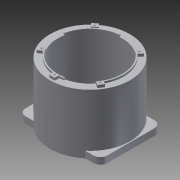
# Autodesk Inventor part: F-mount to CMV12k-V04
Saved by Autodesk Inventor 2015 (Build 190159000, 159)
## iProperties
Created: 2012-09-30
Part Number: F-mount to CMV12k-V04
Document SubType Name: Modeling
Designer: ko
Density: 2.71 g/cm^3
Material: Aluminum-6061
Mass: 114.122 g
Surface Area: 182.607 cm^2
Volume: 42.1113 cm^3
Appearance: Aluminum - Flat
Author: ko
Autodesk Inventor part; units mm, degrees
ref_plane "YZ Plane" through (0, 0, 0) normal (1, 0, 0) x (0, 1, 0)
ref_plane "XZ Plane" through (0, 0, 0) normal (0, 1, 0) x (-1, 0, 0)
ref_plane "Work Plane2" through (0, 0, -4.13) normal (0, 0, 1) x (1, 0, 0)
ref_plane "F-mount flange back plane" through (0, 0, -2.23) normal (0, 0, 1) x (1, 0, 0)
sketch "Sketch2" plane through (0, 0, -4.13) normal (0, 0, 1) x (1, 0, 0)
  circle A0 centre (0, 0) radius 29
  dimension "d2" = 58
  constraints: 1 centre point, 1 coincident
  measures "d2" diameter of A0
sketch "Sketch4" plane through (0, 0, 0) normal (0, 1, 0) x (-1, 0, 0)
  line L0 (0, 0) -> (0, -97.328378) construction
  arc A0 (92.740295, -62.593615) -> (0, 0) centre (0, -100) ccw
  line L1 (29, -4.13) -> (-29, -4.13)
  dimension "d19" = 100
  constraints: 2 end point, 2 point on circle, 1 centre point, 1 point on line, 1 vertical, 2 other
  measures "d19" distance of L0.start A0.centre
ref_plane "Focal plane" through (0, 0, -46.5) normal (0, 0, 1) x (1, 0, 0)
ref_plane "Back origin" through (0, 0, -47.25) normal (0, 0, 1) x (1, 0, 0)
sketch "Sketch3" plane through (0, 0, -46.5) normal (0, 0, 1) x (1, 0, 0)
  line L0 (-24.3, -16.9) -> (22.7, -16.9) construction
  line L1 (22.7, 16.9) -> (-24.3, 16.9) construction
  line L2 (-12.6, 11.4) -> (12.6, 11.4) construction
  line L3 (12.6, 11.4) -> (12.6, -11.4) construction
  line L4 (12.6, -11.4) -> (-12.6, -11.4) construction
  line L5 (-12.6, -11.4) -> (-12.6, 11.4) construction
  line L6 (47.757602, 0) -> (-47.757602, 0) construction
  line L7 (0, 37.75526) -> (0, -37.75526) construction
  line L8 (-0.8, 20.026863) -> (-0.8, -19.024317) construction
  line L9 (22.7, 1.75) -> (20.7, 1.75) construction
  line L10 (20.7, -1.75) -> (22.7, -1.75) construction
  arc A0 (20.7, 1.75) -> (20.7, -1.75) centre (20.7, 0) ccw construction
  line L11 (22.7, 8.9) -> (18.7, 8.9) construction
  line L12 (18.7, 8.9) -> (18.7, 12.9) construction
  line L13 (18.7, 12.9) -> (22.7, 12.9) construction
  line L14 (22.7, 1.75) -> (22.7, 8.9) construction
  line L15 (22.7, 12.9) -> (22.7, 16.9) construction
  line L16 (22.7, -8.9) -> (18.7, -8.9) construction
  line L17 (18.7, -8.9) -> (18.7, -12.9) construction
  line L18 (18.7, -12.9) -> (22.7, -12.9) construction
  line L19 (22.7, -1.75) -> (22.7, -8.9) construction
  line L20 (22.7, -12.9) -> (22.7, -16.9) construction
  line L21 (-24.3, 1.75) -> (-22.3, 1.75) construction
  line L22 (-22.3, -1.75) -> (-24.3, -1.75) construction
  arc A1 (-22.3, -1.75) -> (-22.3, 1.75) centre (-22.3, 0) ccw construction
  line L23 (-24.3, 8.9) -> (-20.3, 8.9) construction
  line L24 (-20.3, 8.9) -> (-20.3, 12.9) construction
  line L25 (-20.3, 12.9) -> (-24.3, 12.9) construction
  line L26 (-24.3, 1.75) -> (-24.3, 8.9) construction
  line L27 (-24.3, 12.9) -> (-24.3, 16.9) construction
  line L28 (-20.3, -8.9) -> (-20.3, -12.9) construction
  line L29 (-24.3, -12.9) -> (-24.3, -16.9) construction
  line L30 (-20.3, -12.9) -> (-24.3, -12.9) construction
  line L31 (-24.3, -8.9) -> (-20.3, -8.9) construction
  line L32 (-24.3, -1.75) -> (-24.3, -8.9) construction
  line L33 (-20.198295, -17.2) -> (-20.43657, -17.382277)
  line L34 (-24.65, -22.15) -> (24.65, -22.15)
  line L35 (29.65, -17.15) -> (29.65, 17.15)
  line L36 (24.65, 22.15) -> (-24.65, 22.15)
  line L37 (-29.65, 17.15) -> (-29.65, -17.15)
  arc A2 (29.65, 17.15) -> (24.65, 22.15) centre (24.65, 17.15) ccw
  arc A3 (24.65, -22.15) -> (29.65, -17.15) centre (24.65, -17.15) ccw
  arc A4 (-29.65, -17.15) -> (-24.65, -22.15) centre (-24.65, -17.15) ccw
  arc A5 (-24.65, 22.15) -> (-29.65, 17.15) centre (-24.65, 17.15) ccw
  line L38 (-24.238989, 12.5) -> (-28.238989, 12.5) construction
  line L39 (-24.3, 12.9) -> (-29.65, 12.9) construction
  line L40 (-27.5, 13.045808) -> (-27.5, 9.045808) construction
  line L41 (28.625588, -12.5) -> (20.569896, -12.5) construction
  line L42 (27.5, -9.401134) -> (27.5, -14.475126) construction
  line L43 (-18.15, 16.9) -> (16.55, 16.9) construction
  line L44 (16.55, 16.9) -> (16.55, -16.9) construction
  line L45 (16.55, -16.9) -> (-18.15, -16.9) construction
  line L46 (-18.15, -16.9) -> (-18.15, 16.9) construction
  point P0 (0, 0)
  point P1 (0, 0)
  point P2 (0, 0)
  point P3 (-20.3, 10.9)
  point P4 (-27.5, 12.5)
  point P5 (27.5, -12.5)
  dimension "d5" = 16.9
  dimension "d6" = 47
  dimension "d7" = 33.8
  dimension "d8" = 25.2
  dimension "d9" = 22.8
  dimension "d10" = 3.5
  dimension "d11" = 2
  dimension "d12" = 4
  dimension "d13" = 4
  dimension "d14" = 4
  dimension "d15" = 24.3
  dimension "d135" = 59.3
  dimension "d136" = 44.3
  dimension "d137" = 5
  dimension "d164" = 55
  dimension "d165" = 25
  dimension "d169" = 34.7
  dimension "d170" = 0
  dimension "d171" = 0
  dimension "d172" = 6.15
  dimension "d173" = 6.2
  constraints: 94 end point, 17 symmetric about line, 12 point on circle, 10 tangent, 9 parallel, 6 centre point, 5 perpendicular, 5 vertical, 4 collinear, 4 horizontal, 4 point on line, 3 equal radius, 3 midpoint, 2 coincident, 8 other
  measures "d5" distance from line of point (0, 0) L0
  measures "d6" distance of L1.start L1.end
  measures "d7" distance of L0.end L1.start
  measures "d8" distance of L2.start L2.end
  measures "d9" distance of L2.end L3.end
  measures "d10" distance between parallel lines of L10 L9
  measures "d11" distance of L9.start L9.end
  measures "d12" distance of L11.end L12.end
  measures "d13" distance of L12.end L13.end
  measures "d14" distance between parallel lines of L1 L13
  measures "d15" distance from line of L7 L0.start
  measures "d135" distance between parallel lines of L37 L35
  measures "d136" distance between parallel lines of L34 L36
  measures "d137" radius of A2
  measures "d164" distance between parallel lines of L42 L40
  measures "d165" distance between parallel lines of L38 L41
  measures "d169" distance of L43.start L43.end
  measures "d170" distance between parallel lines of L0 L45
  measures "d171" distance between parallel lines of L1 L43
  measures "d172" distance between parallel lines of L27 L46
sketch "Sketch6" plane through (0, 0, -46.5) normal (0, 0, 1) x (1, 0, 0)
  line L0 (-0.8, 17.2) -> (-24.3, 17.2)
  line L1 (22.7, 16.9) -> (-24.3, 16.9) construction
  line L2 (-24.3, 12.9) -> (-24.3, 16.9) construction
  arc A0 (-24.3, 17.2) -> (-24.3, 12.775) centre (-24.3, 14.9875) ccw
  line L3 (47.757602, 0) -> (-47.757602, 0) construction
  line L4 (-0.8, 20.026863) -> (-0.8, -19.024317) construction
  line L5 (22.7, 16.9) -> (22.912132, 17.112132) construction
  line L6 (-24.3, 12.775) -> (-20.925, 12.775)
  line L7 (-20.425, 12.275) -> (-20.425, 9.525)
  line L8 (-20.925, 9.025) -> (-24.3, 9.025)
  line L9 (-20.3, 12.9) -> (-24.3, 12.9) construction
  line L10 (-20.3, 8.9) -> (-20.3, 12.9) construction
  line L11 (-24.3, 8.9) -> (-20.3, 8.9) construction
  line L12 (-26.5125, 0) -> (-26.5125, 6.8125)
  arc A1 (-24.3, 9.025) -> (-26.5125, 6.8125) centre (-24.3, 6.8125) ccw
  arc A2 (-20.425, 12.275) -> (-20.925, 12.775) centre (-20.925, 12.275) ccw
  arc A3 (-20.925, 9.025) -> (-20.425, 9.525) centre (-20.925, 9.525) ccw
  line L13 (-0.8, -17.2) -> (-24.3, -17.2)
  line L14 (22.7, -16.9) -> (-24.3, -16.9) construction
  line L15 (-24.3, -12.9) -> (-24.3, -16.9) construction
  arc A4 (-24.3, -12.775) -> (-24.3, -17.2) centre (-24.3, -14.9875) ccw
  line L16 (-24.3, -12.775) -> (-20.925, -12.775)
  line L17 (-20.425, -12.275) -> (-20.425, -9.525)
  line L18 (-20.925, -9.025) -> (-24.3, -9.025)
  line L19 (-20.3, -12.9) -> (-24.3, -12.9) construction
  line L20 (-20.3, -8.9) -> (-20.3, -12.9) construction
  line L21 (-24.3, -8.9) -> (-20.3, -8.9) construction
  line L22 (-26.5125, 0) -> (-26.5125, -6.8125)
  arc A5 (-26.5125, -6.8125) -> (-24.3, -9.025) centre (-24.3, -6.8125) ccw
  arc A6 (-20.925, -12.775) -> (-20.425, -12.275) centre (-20.925, -12.275) ccw
  arc A7 (-20.425, -9.525) -> (-20.925, -9.025) centre (-20.925, -9.525) ccw
  line L23 (-0.8, 17.2) -> (22.7, 17.2)
  line L24 (-24.3, 16.9) -> (22.7, 16.9) construction
  line L25 (22.7, 12.9) -> (22.7, 16.9) construction
  arc A8 (22.7, 12.775) -> (22.7, 17.2) centre (22.7, 14.9875) ccw
  line L26 (-49.357602, 0) -> (46.157602, 0) construction
  line L27 (22.7, 12.775) -> (19.325, 12.775)
  line L28 (18.825, 12.275) -> (18.825, 9.525)
  line L29 (19.325, 9.025) -> (22.7, 9.025)
  line L30 (18.7, 12.9) -> (22.7, 12.9) construction
  line L31 (18.7, 8.9) -> (18.7, 12.9) construction
  line L32 (22.7, 8.9) -> (18.7, 8.9) construction
  line L33 (24.9125, 0) -> (24.9125, 6.8125)
  arc A9 (24.9125, 6.8125) -> (22.7, 9.025) centre (22.7, 6.8125) ccw
  arc A10 (19.325, 12.775) -> (18.825, 12.275) centre (19.325, 12.275) ccw
  arc A11 (18.825, 9.525) -> (19.325, 9.025) centre (19.325, 9.525) ccw
  line L34 (22.7, -12.9) -> (22.7, -16.9) construction
  line L35 (18.7, -8.9) -> (18.7, -12.9) construction
  line L36 (18.825, -12.275) -> (18.825, -9.525)
  arc A12 (18.825, -12.275) -> (19.325, -12.775) centre (19.325, -12.275) ccw
  arc A13 (19.325, -9.025) -> (18.825, -9.525) centre (19.325, -9.525) ccw
  line L37 (18.7, -12.9) -> (22.7, -12.9) construction
  line L38 (22.7, -8.9) -> (18.7, -8.9) construction
  line L39 (19.325, -9.025) -> (22.7, -9.025)
  line L40 (22.7, -12.775) -> (19.325, -12.775)
  arc A14 (22.7, -17.2) -> (22.7, -12.775) centre (22.7, -14.9875) ccw
  line L41 (24.9125, 0) -> (24.9125, -6.8125)
  arc A15 (22.7, -9.025) -> (24.9125, -6.8125) centre (22.7, -6.8125) ccw
  line L42 (-0.8, -17.2) -> (22.7, -17.2)
  line L43 (-24.3, -16.9) -> (22.7, -16.9) construction
  point P0 (0, 0)
  point P1 (-0.8, -20.026863)
  dimension "d37" = 0.3
  dimension "d41" = 0.125
  dimension "d42" = 0.125
  dimension "d43" = 0.125
  dimension "d45" = 2.2125
  dimension "d47" = 0.5
  constraints: 74 end point, 59 symmetric about line, 32 point on circle, 16 centre point, 11 point on line, 8 tangent, 2 equal radius, 1 parallel, 12 other
  measures "d37" distance between parallel lines of L1 L0
  measures "d41" distance between parallel lines of L6 L9
  measures "d42" distance between parallel lines of L10 L7
  measures "d43" distance between parallel lines of L11 L8
  measures "d45" radius of A0
  measures "d47" radius of A2
sketch "Sketch5" plane through (0, 0, -4.13) normal (0, 0, 1) x (1, 0, 0)
  line L0 (29.3063, -36.610535) -> (-29.3063, -36.610535)
  line L1 (-39.3063, -26.610535) -> (-39.3063, 26.610535)
  line L2 (-29.3063, 36.610535) -> (29.3063, 36.610535)
  line L3 (39.3063, 26.610535) -> (39.3063, -26.610535)
  line L4 (39.3063, 36.610535) -> (-39.3063, -36.610535) construction
  arc A0 (-29.3063, 36.610535) -> (-39.3063, 26.610535) centre (-29.3063, 26.610535) ccw
  arc A1 (-39.3063, -26.610535) -> (-29.3063, -36.610535) centre (-29.3063, -26.610535) ccw
  arc A2 (29.3063, -36.610535) -> (39.3063, -26.610535) centre (29.3063, -26.610535) ccw
  arc A3 (39.3063, 26.610535) -> (29.3063, 36.610535) centre (29.3063, 26.610535) ccw
  point P0 (0, 0)
  point P1 (39.3063, -36.610535)
  point P2 (-39.3063, 36.610535)
  point P3 (0, 0)
  dimension "d16" = 78.6126
  dimension "d17" = 73.22107
  dimension "d18" = 10
  constraints: 10 end point, 8 point on circle, 8 point on line, 8 tangent, 4 centre point, 3 equal radius, 2 perpendicular, 1 coincident, 1 horizontal, 1 midpoint, 1 vertical
  measures "d16" distance of point (-39.306, 36.611) L4.start
  measures "d17" distance of L4.start point (39.306, -36.611)
  measures "d18" radius of A0
extrude "Extrusion2" add sketch "Sketch2" against normal up to surface (43.12 mm away)
extrude "Extrusion16" add sketch "Sketch3" along normal blind 4 and the other way blind 0.75
extrude "Extrusion4" cut sketch "Sketch6" against normal blind 4 and the other way blind 2
sketch "Sketch7" plane through (0, 0, -44.5) normal (0, 0, -1) x (-1, 0, 0)
  line L0 (24.3, 17.2) -> (-22.7, 17.2)
  line L1 (-12.6, 11.4) -> (-12.6, -11.4) construction
  line L2 (12.6, 11.4) -> (-12.6, 11.4) construction
  line L3 (-12.6, -11.4) -> (12.6, -11.4) construction
  line L4 (12.6, -11.4) -> (12.6, 11.4) construction
  line L5 (-14.85, 13.4) -> (-14.85, -13.4)
  line L6 (-13.85, -14.4) -> (13.85, -14.4)
  arc A0 (-14.85, -13.4) -> (-13.85, -14.4) centre (-13.85, -13.4) ccw
  arc A1 (14.85, -14.4) -> (14.85002, -14.39998) centre (14.85, -14.39998) ccw
  line L7 (-22.7, 17.2) -> (24.3, 17.2)
  line L8 (-16.55, 16.9) -> (-16.55, -16.9) construction
  line L9 (18.15, -16.9) -> (18.15, 16.9) construction
  line L10 (-22.7, 16.9) -> (24.3, 16.9) construction
  line L11 (24.3, -17.2) -> (-22.7, -17.2) construction
  line L12 (20.925, 12.775) -> (24.3, 12.775)
  line L13 (14.85, -13.4) -> (14.85, 13.4)
  arc A2 (13.85, -14.4) -> (14.85, -13.4) centre (13.85, -13.4) ccw
  line L14 (-13.85, 14.4) -> (13.85, 14.4)
  arc A3 (-13.85, 14.4) -> (-14.85, 13.4) centre (-13.85, 13.4) ccw
  arc A4 (14.85, 13.4) -> (13.85, 14.4) centre (13.85, 13.4) ccw
  line L15 (-14.257107, 13.115379) -> (-42.057107, 13.115379) construction
  line L16 (-42.057107, 13.115379) -> (-42.057107, 34.607732) construction
  line L17 (-42.057107, 34.607732) -> (-14.257107, 34.607732) construction
  line L18 (-14.257107, 34.607732) -> (-14.257107, 13.115379) construction
  line L19 (-13.85, 13.9) -> (13.85, 13.9) construction
  line L20 (14.35, 13.4) -> (14.35, -13.4) construction
  line L21 (13.85, -13.9) -> (-13.85, -13.9) construction
  line L22 (-14.35, -13.4) -> (-14.35, 13.4) construction
  arc A5 (-13.85, 13.9) -> (-14.35, 13.4) centre (-13.85, 13.4) ccw construction
  arc A6 (14.35, 13.4) -> (13.85, 13.9) centre (13.85, 13.4) ccw construction
  arc A7 (13.85, -13.9) -> (14.35, -13.4) centre (13.85, -13.4) ccw construction
  arc A8 (-14.35, -13.4) -> (-13.85, -13.9) centre (-13.85, -13.4) ccw construction
  point P0 (0, 0)
  point P1 (-14.85, 17.2)
  point P2 (-14.85, 14.4)
  point P3 (23.348662, 17.2)
  point P4 (1.637447, 2.242703)
  point P5 (14.35, -13.9)
  point P6 (14.35, 13.9)
  point P7 (-14.35, -13.9)
  dimension "d186" = 1
  dimension "d187" = 1
  dimension "d189" = 1
  dimension "d190" = 27.8
  dimension "d191" = 28.7
  dimension "d192" = 27.8
  dimension "d193" = 14.35
  dimension "d194" = 13.9
  dimension "d195" = 0.5
  dimension "d196" = 0.5
  dimension "d197" = 0.5
  dimension "d198" = 0.5
  dimension "d199" = 0.5
  constraints: 24 end point, 18 point on circle, 17 tangent, 12 point on line, 9 centre point, 4 equal radius, 4 parallel, 4 perpendicular, 2 horizontal
  measures "d186" radius of A0
  measures "d187" radius of A2
  measures "d189" radius of A3
  measures "d190" distance of L16.end L17.end
  measures "d191" distance of point (14.35, -13.9) point (-14.35, -13.9)
  measures "d192" distance of point (14.35, 13.9) point (14.35, -13.9)
  measures "d193" distance from line of point (0, 0) L22
  measures "d194" distance from line of L19 point (0, 0)
  measures "d195" distance between parallel lines of L22 L5
  measures "d196" distance between parallel lines of L19 L14
  measures "d197" distance between parallel lines of L20 L13
  measures "d198" distance between parallel lines of L21 L6
  measures "d199" radius of A5
extrude "Extrusion5" cut sketch "Sketch7" against normal blind 3
sketch "Sketch12" plane through (0, 0, -4.13) normal (0, 0, 1) x (1, 0, 0)
  circle A0 centre (0, 0) radius 27.65 construction
  line L0 (2, -27.577572) -> (2, -24.327572)
  line L1 (-2, -24.327572) -> (-2, -27.577572)
  line L2 (0, -28.225094) -> (0, -23.5) construction
  arc A1 (-2, -24.327572) -> (2, -24.327572) centre (0, 0) ccw
  arc A2 (-2, -27.577572) -> (2, -27.577572) centre (0, 0) ccw
  line L3 (24.202356, -13.370433) -> (21.478722, -11.59721)
  line L4 (18.531302, -14.451327) -> (22.019928, -16.722597)
  line L5 (22.280479, -14.505712) -> (19.693968, -12.821763) construction
  arc A3 (19.296294, -14.949375) -> (21.478722, -11.59721) centre (0, 0) ccw
  line L6 (16.015086, 22.539732) -> (13.364799, 19.329567)
  line L7 (17.030556, 17.48688) -> (19.099683, 19.993114)
  line L8 (18.346958, 22.222797) -> (14.96138, 18.122007) construction
  arc A4 (17.030556, 17.48688) -> (13.945959, 20.033497) centre (0, 0) ccw
  arc A5 (22.019928, -16.722597) -> (24.202356, -13.370433) centre (0, 0) ccw
  arc A6 (19.099683, 19.993114) -> (16.015086, 22.539732) centre (0, 0) ccw
  line L9 (-24.202356, -13.370433) -> (-20.71373, -11.099162)
  line L10 (-19.296294, -14.949375) -> (-22.019928, -16.722597)
  arc A7 (-21.478722, -11.59721) -> (-19.296294, -14.949375) centre (0, 0) ccw
  line L11 (-22.280479, -14.505712) -> (-19.693968, -12.821763) construction
  line L12 (-16.015086, 22.539732) -> (-13.945959, 20.033497)
  line L13 (-17.030556, 17.48688) -> (-19.099683, 19.993114)
  arc A8 (-13.945959, 20.033497) -> (-17.030556, 17.48688) centre (0, 0) ccw
  line L14 (-18.346958, 22.222797) -> (-14.96138, 18.122007) construction
  arc A9 (-24.202356, -13.370433) -> (-22.019928, -16.722597) centre (0, 0) ccw
  arc A10 (-16.015086, 22.539732) -> (-19.099683, 19.993114) centre (0, 0) ccw
  line L15 (4.984614, -22.96527) -> (5.17756, -23.854217)
  line L16 (-23.018236, 4.734008) -> (-23.909233, 4.917253)
  line L17 (-2.18895, 24.311299) -> (-2.107377, 23.405319)
  arc A11 (18.531302, -14.451327) -> (13.364799, 19.329567) centre (0, 0) ccw
  arc A12 (19.296294, -14.949375) -> (13.945959, 20.033497) centre (0, 0) ccw
  arc A13 (-2.18895, 24.311299) -> (-23.909233, 4.917253) centre (0, 0) ccw
  arc A14 (-21.478722, -11.59721) -> (5.17756, -23.854217) centre (0, 0) ccw
  arc A15 (-2.107377, 23.405319) -> (-23.018236, 4.734008) centre (0, 0) ccw
  arc A16 (-20.71373, -11.099162) -> (4.984614, -22.96527) centre (0, 0) ccw
  line L18 (-21.478722, -11.59721) -> (-20.71373, -11.099162)
  line L19 (13.945959, 20.033497) -> (13.364799, 19.329567)
  line L20 (18.531302, -14.451327) -> (19.296294, -14.949375)
  line L21 (-21.478722, -11.59721) -> (-24.202356, -13.370433)
  circle A17 centre (0, 0) radius 23.5
  circle A18 centre (0, 0) radius 25.5 construction
  point P0 (-21.370051, -13.912977)
  point P1 (21.370051, -13.912977)
  point P2 (16.234688, 19.664305)
  point P3 (-16.234688, 19.664305)
  point P4 (0, -25.5)
  dimension "d73" = 4
  dimension "d74" = 55.3
  dimension "d76" = 3.25
  dimension "d77" = 4
  dimension "d78" = 3.25
  dimension "d79" = 4
  dimension "d90" = 23.5
  dimension "d91" = 3.25
  dimension "d92" = 16
  dimension "d93" = 16
  dimension "d94" = 16
  dimension "d99" = 47
  dimension "d105" = 113.868
  dimension "d106" = 79.0856
  dimension "d107" = 51
  constraints: 47 point on circle, 44 end point, 19 centre point, 17 point on line, 12 coincident, 12 symmetric about line, 4 concentric, 2 collinear, 1 parallel, 1 vertical, 7 other
  measures "d73" distance between parallel lines of L1 L0
  measures "d74" diameter of A0
  measures "d76" distance of L0.start L0.end
  measures "d77" distance between parallel lines of L4 L3
  measures "d78" distance of L3.start L3.end
  measures "d79" distance between parallel lines of L7 L6
  measures "d90" radius of A16
  measures "d91" distance of L7.start L7.end
  measures "d92" distance of L6.end L17.end
  measures "d93" distance of L9.end L16.start
  measures "d94" distance of L4.start L15.start
  measures "d99" diameter of A17
  measures "d105" angle of L5 L11
  measures "d106" angle of L8 L14
  measures "d107" diameter of A18
extrude "Extrusion10" add sketch "Sketch12" along normal up to surface (1.9 mm away) contours A2 L1 A1 L0 | L10 A9 L9 A7 | A3 L3 A5 L4 | L13 A10 L12 A8 | A4 L6 A6 L7
extrude "Extrusion13" add sketch "Sketch12" along normal blind 1.3 contours A1 A14 A7 L9 A16 L15 | A11 L6 A4 A12 A3 L4 | L16 A13 A8 L17 A15
extrude "Extrusion15" cut sketch "Sketch12" against normal up to surface (37.37 mm away) contours A16 A17 A15 A11
sketch "Sketch15" plane through (0, 0, -2.23) normal (0, 0, 1) x (1, 0, 0)
  circle A0 centre (0, 0) radius 25.5 construction
  line L0 (-18.346958, 22.222797) -> (-14.96138, 18.122007) construction
  line L1 (18.346958, 22.222797) -> (14.96138, 18.122007) construction
  line L2 (0, -28.225094) -> (0, -23.5) construction
  line L3 (22.280479, -14.505712) -> (19.693968, -12.821763) construction
  line L4 (29.3063, -36.610535) -> (-29.3063, -36.610535)
  line L5 (-29.3063, -36.610535) -> (29.3063, -36.610535)
  line L6 (-22.280479, -14.505712) -> (-19.693968, -12.821763) construction
  point P0 (-16.234688, 19.664305)
  point P1 (0, -25.5)
  point P2 (-21.370051, -13.912977)
  point P3 (21.370051, -13.912977)
  point P4 (16.234688, 19.664305)
hole "Hole1" at (-16.234688, 19.664305, -2.23) at (16.234688, 19.664305, -2.23) at (21.370051, -13.912977, -2.23) at (0, -25.5, -2.23) at (-21.370051, -13.912977, -2.23) direction (0, 0, -1) diameter 1 depth 3 tip angle 118
thread "Thread1" size "M2x0.4" class "6H" standard "ANSI Metric M Profile" full length
thread "Thread2" size "M2x0.4" class "6H" standard "ANSI Metric M Profile" full length
thread "Thread3" size "M2x0.4" class "6H" standard "ANSI Metric M Profile" full length
thread "Thread4" size "M2x0.4" class "6H" standard "ANSI Metric M Profile" full length
thread "Thread5" size "M2x0.4" class "6H" standard "ANSI Metric M Profile" full length
sketch "Sketch17" plane through (0, 0, -47.25) normal (0, 0, 1) x (1, 0, 0)
  line L0 (-12.727748, 0) -> (10.95493, 0) construction
  point P0 (0, 0)
  point P1 (27.5, -12.5)
  point P2 (-27.5, 12.5)
  point P3 (27.5, 12.5)
  point P4 (-27.5, -12.5)
  dimension "d168" = 25
  constraints: 2 end point, 2 symmetric about line, 1 horizontal
  measures "d168" distance of point (27.5, -12.5) point (27.5, 12.5)
hole "Hole2" [suppressed]
thread "Thread6" size "M2x0.4" class "6H" standard "ANSI Metric M Profile" full length
thread "Thread7" size "M2x0.4" class "6H" standard "ANSI Metric M Profile" full length
hole "Hole3" at (20.7, 0, -46.5) at (-22.3, 0, -46.5) direction (0, 0, 1) diameter 1 end through all
thread "Thread8" size "M2x0.4" class "6H" standard "ANSI Metric M Profile" full length
thread "Thread9" size "M2x0.4" class "6H" standard "ANSI Metric M Profile" full length
equation "\"Die_tickness\" = 0.75"
body "Solid1"
